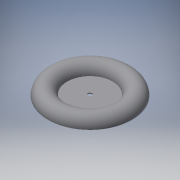
# Autodesk Inventor part: Toroid
Saved by Autodesk Inventor 2019 (Build 230136000, 136)
## iProperties
Created: 2020-12-21
Part Number: Toroid
Material: Типовые
Document SubType Name: Modeling
Designer: Dazer
Density: 1 g/cm^3
Appearance: По умолчанию
Author: Dazer
Autodesk Inventor part; units mm, degrees
ref_plane "YZ Plane" through (0, 0, 0) normal (1, 0, 0) x (0, 1, 0)
ref_plane "XZ Plane" through (0, 0, 0) normal (0, 1, 0) x (-1, 0, 0)
ref_plane "XY Plane" through (0, 0, 0) normal (0, 0, 1) x (1, 0, 0)
sketch "Эскиз1" plane through (0, 0, 0) normal (1, 0, 0) x (0, 1, 0)
  line L0 (0, -3.5) -> (1.4, -3.5)
  arc A0 (0, -65) -> (1.4, -35.0655) centre (0, -50) ccw
  line L1 (0, 0) -> (3.7667, 0)
  line L2 (0, -3.5) -> (0, -35)
  line L3 (1.4, -3.5) -> (1.4, -35.0655)
  arc A1 (0, -63.6) -> (0, -36.4) centre (0, -50) ccw
  line L4 (0, -35) -> (0, -36.4)
  line L5 (0, -63.6) -> (0, -65)
  dimension "d0" = 3.5
  dimension "d1" = 1.4
  constraints: 12 end point, 4 point on circle, 2 centre point, 2 point on line, 2 vertical, 1 coincident, 1 horizontal, 1 parallel
  measures "d0" distance of L1.start L0.start
  measures "d1" distance of L0.start L0.end
revolve "Вращение1" add sketch "Эскиз1" angle 360 about axis through (0, 0, 0) along (0, 1, 0)
sketch "Эскиз2" plane through (0, 0, 0) normal (0, -1, 0) x (1, 0, 0)
  circle A0 centre (0, 0) radius 36.4 projected
  line L0 (0.7, -36.2) -> (-0.7, -36.2)
  line L1 (0.7, -63.8) -> (-0.7, -63.8)
  line L2 (-0.7, -63.8) -> (-0.7, -36.2)
  line L3 (0.7, -36.2) -> (0.7, -63.8)
  dimension "d9" = 1.4
  constraints: 8 end point, 1 parallel, 1 perpendicular
  measures "d9" distance of L0.start L0.end
extrude "Выдавливание1" add sketch "Эскиз2" against normal through all contours L2 L0 L3 A0 | A0 L3 L1 L2 picked at (-0.0778, -36.2664)
pattern_circular "Круговой массив1" count 10 over 360 about axis through (0, 0.7, 0) along (0, -1, 0) of "Выдавливание1"
